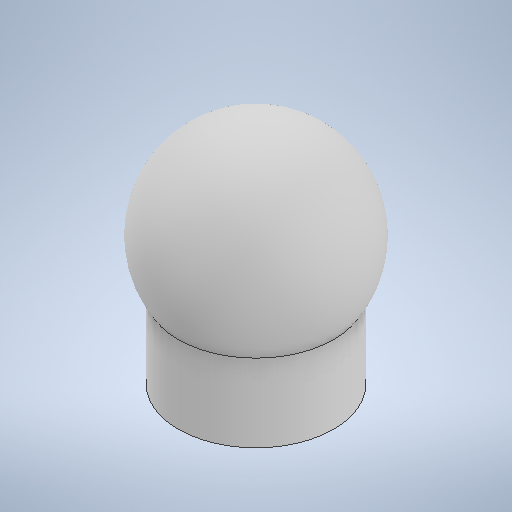
# Autodesk Inventor part: Test2
Saved by Autodesk Inventor 2026.2 (Build 302298010, 298A)
## iProperties
Created: 2026-05-09
Part Number: Test2
Material: Generic
Document SubType Name: Modeling
Designer: piete
Density: 1 g/cm^3
Appearance: Default
Author: piete
Autodesk Inventor part; units mm, degrees
ref_plane "YZ Plane" through (0, 0, 0) normal (1, 0, 0) x (0, 1, 0)
ref_plane "XZ Plane" through (0, 0, 0) normal (0, 1, 0) x (-1, 0, 0)
ref_plane "XY Plane" through (0, 0, 0) normal (0, 0, 1) x (1, 0, 0)
sketch "Sketch1" plane through (0, 0, 0) normal (0, 1, 0) x (-1, 0, 0)
  circle A0 centre (0, 0) radius 10
  dimension "d0" = 20
  constraints: 1 centre point, 1 coincident
  measures "d0" diameter of A0
extrude "Extrusion1" add sketch "Sketch1" along normal blind 10
sketch "Sketch2" plane through (0, 0, 0) normal (1, 0, 0) x (0, 1, 0)
  line L0 (10, -10) -> (10, 10) projected
  line L1 (10, 0) -> (10, 12)
  line L2 (10, 0) -> (10, -12)
  circle A0 centre (10, -10) radius 12
  circle A1 centre (10, 10) radius 12
  circle A2 centre (16.6332, 0) radius 12
  line L3 (30.6793, 0) -> (0, 0)
  point P0 (28.6332, 0)
  point P1 (4.6332, 0)
  dimension "d5" = 24
  dimension "d6" = 24
  dimension "d3" = 12
  dimension "d4" = 12
  dimension "d7" = 24
  constraints: 6 end point, 2 coincident, 1 centre point, 1 collinear, 1 horizontal, 1 midpoint, 1 point on line, 6 other
  measures "d3" distance of L1.start L1.end
  measures "d4" distance of L1.start L2.end
  measures "d7" diameter of A2
revolve "Revolution1" add sketch "Sketch2" angle 360 about axis through (0, 30.6793, 0) along (0, -1, 0) picked at (16.5939, 5.7519) picked at (22.6926, 2.0814) contours L3 A2 A0 L0 | L0 A0 L3 | A0 L0 A2 A1 | A1 A2 L3 | A0 A2 L0
body "Solid1"
